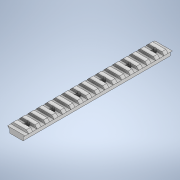
# Autodesk Inventor part: Picatinny Rail
Saved by Autodesk Inventor 2021 (Build 250183000, 183)
## iProperties
Created: 2024-08-02
Part Number: Picatinny Rail
Material: Generic
Document SubType Name: Modeling
Designer: Lukas
Density: 1 g/cm^3
Appearance: Default
Author: Lukas
Autodesk Inventor part; units mm, degrees
ref_plane "YZ Plane" through (0, 0, 0) normal (1, 0, 0) x (0, 1, 0)
ref_plane "XZ Plane" through (0, 0, 0) normal (0, 1, 0) x (-1, 0, 0)
ref_plane "XY Plane" through (0, 0, 0) normal (0, 0, 1) x (1, 0, 0)
sketch "Sketch1" plane through (0, 0, 0) normal (0, 0, 1) x (1, 0, 0)
  line L0 (-7.835, 0) -> (7.835, 0)
  line L1 (7.835, 0) -> (7.835, 3.78)
  line L2 (7.835, 3.78) -> (10.605, 6.55)
  line L3 (10.605, 6.55) -> (7.835, 9.32)
  line L4 (-7.835, 9.32) -> (-10.605, 6.55)
  line L5 (-10.605, 6.55) -> (-7.835, 3.78)
  line L6 (-7.835, 3.78) -> (-7.835, 0)
  line L7 (-7.835, 9.32) -> (7.835, 9.32)
  point P0 (0, 0)
  point P1 (0, 0)
  dimension "d0" = 15.67
  dimension "d1" = 21.21
  dimension "d2" = 3.78
  constraints: 16 end point, 5 perpendicular, 2 coincident, 2 horizontal, 2 horizontal alignment, 1 midpoint, 1 point on line, 1 vertical
  measures "d0" distance of L4.start L3.end
  measures "d1" distance of L2.end L4.end
  measures "d2" distance of L5.end L0.start
extrude "Extrusion1" add sketch "Sketch1" along normal blind 174
sketch "Sketch3" plane through (-7.835, 9.32, 0) normal (0, 1, 0) x (1, 0, 0)
  circle A0 centre (7.835, -12.625) radius 1.6
  circle A1 centre (7.835, -12.625) radius 3
  line L0 (15.67, 0) -> (0, 0) projected
  point P0 (7.835, 0)
  point P1 (7.835, 0)
  dimension "d19" = 3.2
  dimension "d20" = 6
  dimension "d21" = 12.625
  constraints: 2 centre point, 1 coincident, 1 midpoint, 1 vertical alignment
  measures "d19" diameter of A0
  measures "d20" diameter of A1
  measures "d21" distance from line of L0 A0.centre
extrude "Extrusion4" cut sketch "Sketch3" against normal through all contours A0
extrude "Extrusion5" cut sketch "Sketch3" against normal blind 7.32
sketch "Sketch2" plane through (0, 0, 0) normal (1, 0, 0) x (0, 1, 0)
  line L0 (6.55, 0) -> (9.32, 0) projected
  line L1 (6.32, 0) -> (10.32, 0)
  line L2 (10.32, 0) -> (10.32, 5.25)
  line L3 (10.32, 5.25) -> (6.32, 5.25)
  line L4 (6.32, 5.25) -> (6.32, 0)
  line L5 (0, 0) -> (0, 174) projected
  dimension "d9" = 4
  dimension "d10" = 5.25
  dimension "d13" = 10.32
  constraints: 8 end point, 2 parallel, 1 horizontal, 1 horizontal alignment, 1 perpendicular
  measures "d9" distance of L2.end L3.end
  measures "d10" distance of L1.end L2.end
  measures "d13" distance between parallel lines of L5 L2
extrude "Extrusion3" cut sketch "Sketch2" along normal through all both and the other way through all
pattern_linear "Rectangular Pattern1" count 20 spacing 10 along (0, 0, 1) of "Extrusion3"
pattern_linear "Rectangular Pattern2" count 7 spacing 30 along (0, 0, 1) of "Extrusion5", "Extrusion4"
body "Solid1"
